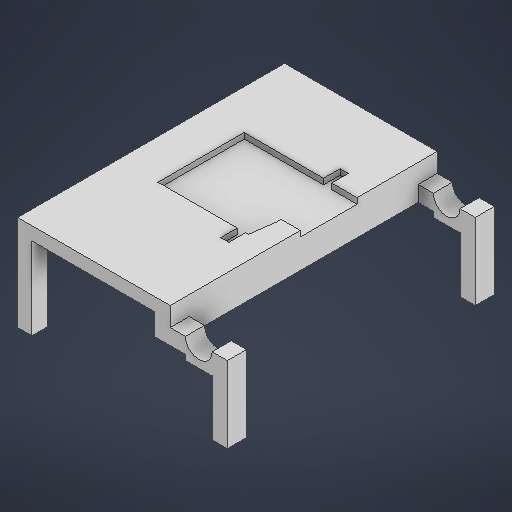
# Autodesk Inventor part: servo_sandboxv3
Saved by Autodesk Inventor 2026.1 (Build 301233020, 233B)
## iProperties
Created: 2026-02-13
Part Number: servo_sandboxv3
Material: Generic
Document SubType Name: Modeling
Designer: Dylan
Density: 1 g/cm^3
Appearance: Default
Author: Dylan
Autodesk Inventor part; units mm, degrees
ref_plane "YZ Plane" through (0, 0, 0) normal (1, 0, 0) x (0, 1, 0)
ref_plane "XZ Plane" through (0, 0, 0) normal (0, 1, 0) x (-1, 0, 0)
ref_plane "XY Plane" through (0, 0, 0) normal (0, 0, 1) x (1, 0, 0)
sketch "Sketch1" plane through (0, 0, 0) normal (0, 1, 0) x (-1, 0, 0)
  line L0 (-40, 0) -> (-40, -60)
  line L1 (0, -60) -> (0, 0)
  line L2 (-40, -60) -> (-55, -60)
  line L3 (-55, -60) -> (-55, -65)
  line L4 (-55, -65) -> (0, -65)
  line L5 (0, -65) -> (0, -60)
  line L6 (-40, 0) -> (-55, 0)
  line L7 (-55, 0) -> (-55, 5)
  line L8 (-55, 5) -> (0, 5)
  line L9 (0, 5) -> (0, 0)
  constraints: 20 end point, 5 parallel, 2 horizontal, 2 perpendicular
extrude "Extrusion1" add sketch "Sketch1" along normal blind 25
sketch "Sketch2" plane through (0, 25, 0) normal (0, 1, 0) x (1, 0, 0)
  line L0 (55, 0) -> (40, 0) projected
  line L1 (40, 0) -> (55, 0)
  line L2 (55, 0) -> (55, -5)
  line L3 (55, -5) -> (40, -5)
  line L4 (40, -5) -> (40, 0)
  line L5 (40, 0) -> (40, 60) projected
  line L6 (55, 60) -> (55, 65) projected
  line L7 (40, 60) -> (55, 60)
  line L8 (55, 60) -> (55, 65)
  line L9 (55, 65) -> (40, 65)
  line L10 (40, 65) -> (40, 60)
  point P0 (0, 0)
  constraints: 16 end point, 4 parallel, 2 horizontal, 2 perpendicular
extrude "Extrusion2" cut sketch "Sketch2" against normal blind 5
sketch "Sketch3" plane through (0, 0, 5) normal (0, 0, 1) x (1, 0, 0)
  line L0 (55, 20) -> (40, 20) projected
  circle A0 centre (47.5, 20) radius 3.5
  point P0 (0, 0)
  dimension "d10" = 7
  constraints: 1 centre point, 1 midpoint
  measures "d10" diameter of A0
extrude "Extrusion3" cut sketch "Sketch3" against normal through all
sketch "Sketch4" plane through (0, 25, 0) normal (0, 1, 0) x (1, 0, 0)
  line L0 (40, 0) -> (40, 60) projected
  line L1 (40, 44.0004) -> (40, 29.1004)
  line L2 (40, 29.1004) -> (35, 29.1004)
  line L3 (35, 29.1004) -> (35, 28.1004)
  line L4 (31.2, 48.3504) -> (31.2, 44.0004)
  line L5 (31.2, 44.0004) -> (10.4, 44.0004)
  line L6 (10.4, 44.0004) -> (10.4, 21.4004)
  line L7 (10.4, 21.4004) -> (31.2, 21.4004)
  line L8 (31.2, 21.4004) -> (31.2, 17.0504)
  line L9 (34.1, 21.4004) -> (35, 28.1004)
  line L10 (31.2, 17.0504) -> (33.35, 17.0504)
  line L11 (33.35, 17.0504) -> (33.35, 21.4004)
  line L12 (33.35, 21.4004) -> (34.1, 21.4004)
  line L13 (31.2, 48.3504) -> (33.35, 48.3504)
  line L14 (33.35, 48.3504) -> (33.35, 44.0004)
  line L15 (33.35, 44.0004) -> (40, 44.0004)
  point P0 (0, 0)
  dimension "d13" = 14.9
  dimension "d14" = 5
  dimension "d15" = 1
  dimension "d19" = 20.8
  dimension "d20" = 22.6
  dimension "d21" = 20.8
  dimension "d32" = 2.15
  dimension "d33" = 2.15
  constraints: 30 end point, 5 perpendicular, 5 point on line, 2 horizontal, 2 vertical
  measures "d13" distance of L1.start L1.end
  measures "d14" distance of L1.end L2.end
  measures "d15" distance of L2.end L3.end
  measures "d19" distance of L4.end L5.end
  measures "d20" distance of L5.end L6.end
  measures "d21" distance of L6.end L7.end
  measures "d32" distance of L8.end L10.end
  measures "d33" distance of L4.start L13.end
extrude "Extrusion4" cut sketch "Sketch4" against normal blind 1.5
sketch "Sketch5" plane through (0, 0, 5) normal (0, 0, 1) x (1, 0, 0)
  line L0 (55, 0) -> (0, 0) projected
  line L1 (44.0382, 15.8995) -> (35.8479, 15.8995)
  line L2 (3.7342, 15.8995) -> (3.7342, 0)
  line L3 (3.7342, 0) -> (51, 0)
  line L4 (51, 0) -> (51, 14.5037)
  line L5 (51, 14.5037) -> (44.0382, 14.5037)
  line L6 (44.0382, 14.5037) -> (44.0382, 15.8995)
  line L7 (3.7342, 15.8995) -> (3.7342, 21.5553)
  line L8 (3.7342, 21.5553) -> (35.8479, 21.5553)
  line L9 (35.8479, 21.5553) -> (35.8479, 15.8995)
  constraints: 18 end point, 5 perpendicular, 2 parallel, 1 horizontal, 1 point on line, 1 vertical
extrude "Extrusion5" cut sketch "Sketch5" against normal through all
sketch "Sketch9" plane through (0, 0, -65) normal (-1, 0, 0) x (0, 0, 1)
  line L0 (70, 0) -> (65, 0) projected
  line L1 (5.02, 21.545) -> (65.98, 21.545)
  line L2 (65.98, 21.545) -> (65.98, 0)
  line L3 (65.98, 0) -> (5.02, 0)
  line L4 (5.02, 0) -> (5.02, 21.545)
  dimension "d29" = 60.96
  constraints: 8 end point, 2 parallel, 1 horizontal, 1 perpendicular, 1 point on line
  measures "d29" distance of L2.end L3.end
extrude "Extrusion6" cut sketch "Sketch9" against normal blind 10
body "Solid1"
